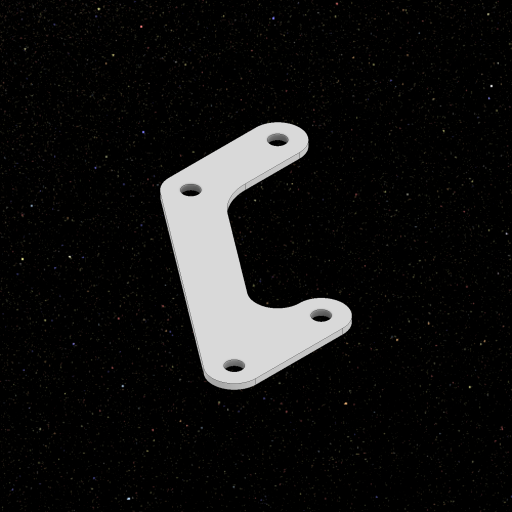
# Autodesk Inventor part: gusset
Saved by Autodesk Inventor 2024 (Build 280153000, 153)
## iProperties
Created: 2024-02-24
Part Number: gusset
Material: Generic
Document SubType Name: Modeling
Designer: Averey Ku
Density: 1 g/cm^3
Appearance: Default
Author: Averey Ku
Autodesk Inventor part; units mm, degrees
ref_plane "YZ Plane" through (0, 0, 0) normal (1, 0, 0) x (0, 1, 0)
ref_plane "XZ Plane" through (0, 0, 0) normal (0, 1, 0) x (-1, 0, 0)
ref_plane "XY Plane" through (0, 0, 0) normal (0, 0, 1) x (1, 0, 0)
sketch "main" plane through (0, 0, 0) normal (0, 0, 1) x (1, 0, 0)
  circle A0 centre (-23.0544, 32.6599) radius 2.1844
  circle A1 centre (-23.0544, 7.2599) radius 2.1844
  circle A2 centre (27.7456, -5.4401) radius 2.1844
  arc A3 (34.0956, -5.4401) -> (31.5556, -0.3601) centre (27.7456, -5.4401) ccw
  arc A4 (21.3956, -14.9651) -> (16.3156, -4.8051) centre (8.6956, -14.9651) ccw
  line L0 (-6.5444, 12.3399) -> (16.3156, -4.8051)
  line L1 (-16.7044, 7.2599) -> (-16.7044, 7.2599)
  arc A5 (-6.5444, 12.3399) -> (-16.7044, 7.2599) centre (-10.3544, 7.2599) ccw
  arc A6 (-29.4044, 7.2599) -> (-16.7044, 7.2599) centre (-23.0544, 7.2599) ccw
  line L2 (31.5556, -0.3601) -> (-19.2444, 37.7399)
  line L3 (-29.4044, 32.6599) -> (-29.4044, 7.2599)
  arc A7 (-19.2444, 37.7399) -> (-29.4044, 32.6599) centre (-23.0544, 32.6599) ccw
  line L4 (34.0956, -5.4401) -> (34.0956, -30.8401)
  line L5 (21.3956, -14.9651) -> (21.3956, -30.8401)
  circle A8 centre (27.7456, -30.8401) radius 2.1844
  arc A9 (21.3956, -30.8401) -> (34.0956, -30.8401) centre (27.7456, -30.8401) ccw
  point P0 (4.3446, 0.8511)
  dimension "d0" = 6.35
  dimension "d1" = 12.7
  measures "d0" radius of A5
  measures "d1" radius of A4
sketch "Sketch1" plane through (0, 0, 0) normal (0, 1, 0) x (-1, 0, 0)
  circle A0 centre (0, 25.4) radius 2.1844
  circle A1 centre (0, 0) radius 2.1844
  circle A2 centre (50.8, -12.7) radius 2.1844
  arc A3 (57.15, -12.7) -> (54.61, -7.62) centre (50.8, -12.7) ccw
  arc A4 (44.45, -22.225) -> (39.37, -12.065) centre (31.75, -22.225) ccw
  line L0 (16.51, 5.08) -> (39.37, -12.065)
  line L1 (6.35, 0) -> (6.35, 0)
  arc A5 (16.51, 5.08) -> (6.35, 0) centre (12.7, 0) ccw
  arc A6 (-6.35, 0) -> (6.35, 0) centre (0, 0) ccw
  line L2 (54.61, -7.62) -> (3.81, 30.48)
  line L3 (-6.35, 25.4) -> (-6.35, 0)
  arc A7 (3.81, 30.48) -> (-6.35, 25.4) centre (0, 25.4) ccw
  line L4 (57.15, -12.7) -> (57.15, -38.1)
  line L5 (44.45, -22.225) -> (44.45, -38.1)
  circle A8 centre (50.8, -38.1) radius 2.1844
  arc A9 (44.45, -38.1) -> (57.15, -38.1) centre (50.8, -38.1) ccw
  constraints: 1 other
extrude "Extrusion1" add sketch "Sketch1" along normal blind 1.5875
body "Solid1"
